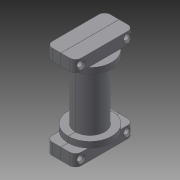
# Autodesk Inventor part: bearing v2
Saved by Autodesk Inventor 2015 (Build 190159000, 159)
## iProperties
Created: 2019-01-15
Part Number: bearing v2
Material: Generic
Document SubType Name: Modeling
Designer: Toby
Density: 1 g/cm^3
Appearance: Default
Author: Toby
Autodesk Inventor part; units mm, degrees
ref_plane "YZ Plane" through (0, 0, 0) normal (1, 0, 0) x (0, 1, 0)
ref_plane "XZ Plane" through (0, 0, 0) normal (0, 1, 0) x (-1, 0, 0)
ref_plane "XY Plane" through (0, 0, 0) normal (0, 0, 1) x (1, 0, 0)
sketch "Sketch1" plane through (0, 0, 0) normal (0, 0, 1) x (1, 0, 0)
  circle A0 centre (0, 0) radius 2.75
  circle A1 centre (0, 0) radius 5
  dimension "d0" = 5.5
  dimension "d1" = 10
  constraints: 2 centre point, 2 coincident
  measures "d0" diameter of A0
  measures "d1" diameter of A1
extrude "Extrusion1" add sketch "Sketch1" along normal blind 20
sketch "Sketch2" plane through (0, 0, 20) normal (0, 0, 1) x (1, 0, 0)
  circle A0 centre (0, 0) radius 7.5
  dimension "d4" = 15
  constraints: 1 centre point, 1 coincident
  measures "d4" diameter of A0
extrude "Extrusion2" add sketch "Sketch2" along normal blind 2
sketch "Sketch3" plane through (0, 0, 0) normal (0, 0, -1) x (-1, 0, 0)
  circle A0 centre (0, 0) radius 2.75
  circle A1 centre (0, 0) radius 7.5
  constraints: 2 centre point, 2 coincident
extrude "Extrusion3" add sketch "Sketch3" along normal blind 2
sketch "Sketch4" plane through (0, 0, -2) normal (0, 0, -1) x (-1, 0, 0)
  line L0 (-7.5, -10) -> (7.5, -10)
  line L1 (7.5, -10) -> (7.5, 10)
  line L2 (7.5, 10) -> (-7.5, 10)
  line L3 (-7.5, 10) -> (-7.5, -10)
  circle A0 centre (0, 0) radius 2.75
  dimension "d9" = 10
  dimension "d10" = 10
  dimension "d11" = 7.5
  dimension "d12" = 7.5
  constraints: 8 end point, 2 parallel, 1 centre point, 1 coincident, 1 horizontal, 1 perpendicular
  measures "d9" distance from line of point (0, 0) L0
  measures "d10" distance from line of L2 point (0, 0)
  measures "d11" distance from line of point (0, 0) L3
  measures "d12" distance from line of L1 point (0, 0)
extrude "Extrusion4" add sketch "Sketch4" along normal blind 4
sketch "Sketch5" plane through (0, 0, -6) normal (0, 0, -1) x (-1, 0, 0)
  line L0 (7.5, 10) -> (-7.5, 10) projected
  line L1 (-7.5, -10) -> (-5, -10)
  line L2 (-5, -10) -> (-5, 10)
  line L3 (-5, 10) -> (-7.5, 10)
  line L4 (-7.5, 10) -> (-7.5, -10)
  line L5 (7.5, -10) -> (5, -10)
  line L6 (5, -10) -> (5, 10)
  line L7 (5, 10) -> (7.5, 10)
  line L8 (7.5, 10) -> (7.5, -10)
  point P0 (0, 0)
  dimension "d15" = 10
  dimension "d16" = 2.5
  constraints: 16 end point, 4 parallel, 2 horizontal, 2 perpendicular, 2 point on line
  measures "d15" distance between parallel lines of L6 L2
  measures "d16" distance between parallel lines of L4 L2
extrude "Extrusion5" cut sketch "Sketch5" against normal blind 4
sketch "Sketch6" plane through (5, -10, -6) normal (1, 0, 0) x (0, 0, -1)
  line L0 (0, 0) -> (-4, 0) projected
  line L1 (0, 20) -> (-4, 20) projected
  line L2 (-4, 15.5902) -> (-4, 20) projected
  line L3 (-4, 0) -> (-4, 4.4098) projected
  point P0 (-6, 10)
  point P1 (-2, 2)
  point P2 (-2, 18)
  dimension "d19" = 2
  dimension "d20" = 2
  dimension "d21" = 2
  dimension "d22" = 2
  measures "d19" distance from line of L0 point (-2, 2)
  measures "d20" distance from line of L1 point (-2, 18)
  measures "d21" distance from line of L2 point (-2, 18)
  measures "d22" distance from line of L3 point (-2, 2)
hole "Hole1" at (5, -8, -4) at (5, 8, -4) direction (-1, 0, 0) diameter 2 depth 10 tip angle 118 countersink diameter 3 countersink angle 90
sketch "Sketch7" plane through (0, 0, 22) normal (0, 0, 1) x (1, 0, 0)
  line L0 (5, 10) -> (-5, 10)
  line L1 (-5, 10) -> (-5, -10)
  line L2 (-5, -10) -> (5, -10)
  line L3 (5, -10) -> (5, 10)
  point P0 (0, 0)
  constraints: 8 end point, 2 parallel, 1 horizontal, 1 perpendicular
extrude "Extrusion6" add sketch "Sketch7" along normal blind 4
sketch "Sketch8" plane through (5, -10, 22) normal (1, 0, 0) x (0, 0, -1)
  line L0 (0, 20) -> (-4, 20) projected
  line L1 (0, 0) -> (-4, 0) projected
  point P0 (22, 10)
  point P1 (-2, 18)
  point P2 (-2, 2)
  dimension "d32" = 2
  dimension "d33" = 2
  measures "d32" distance from line of L0 point (-2, 18)
  measures "d33" distance from line of L1 point (-2, 2)
hole "Hole2" at (5, 8, 24) at (5, -8, 24) direction (-1, 0, 0) diameter 2 depth 10 tip angle 118 countersink diameter 3 countersink angle 90
fillet "Fillet1" radius 2 8 edges at (5, -10, -4) (-5, -10, -4) (5, -10, 24) (-5, -10, 24) (5, 10, -4) (-5, 10, -4) (-5, 10, 24) (5, 10, 24)
sketch "Sketch9" plane through (0, 0, 26) normal (0, 0, 1) x (1, 0, 0)
  line L0 (0.01, 10.2049) -> (-0.01, 10.2049)
  line L1 (-0.01, 10.2049) -> (-0.01, -10.4514)
  line L2 (-0.01, -10.4514) -> (0.01, -10.4514)
  line L3 (0.01, -10.4514) -> (0.01, 10.2049)
  point P0 (0, 0)
  dimension "d42" = 0.01
  dimension "d43" = 0.01
  constraints: 8 end point, 2 parallel, 1 horizontal, 1 perpendicular
  measures "d42" distance from line of point (0, 0) L3
  measures "d43" distance from line of point (0, 0) L1
extrude "Extrusion7" cut sketch "Sketch9" against normal blind 50
body "Solid1"
